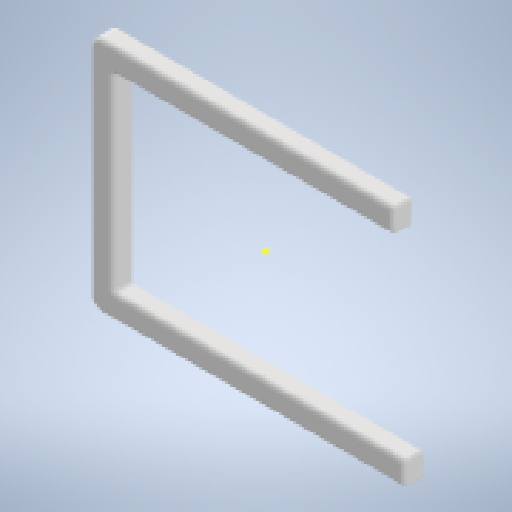
# Autodesk Inventor part: Top_Left
Saved by Autodesk Inventor 2023 (Build 270158000, 158)
## iProperties
Created: 2022-11-13
Part Number: Top_Left
Material: Generic
Document SubType Name: Modeling
Designer: reide
Density: 1 g/cm^3
Appearance: Default
Author: reide
Autodesk Inventor part; units mm, degrees
ref_plane "YZ Plane" through (0, 0, 0) normal (1, 0, 0) x (0, 1, 0)
ref_plane "XZ Plane" through (0, 0, 0) normal (0, 1, 0) x (-1, 0, 0)
ref_plane "XY Plane" through (0, 0, 0) normal (0, 0, 1) x (1, 0, 0)
sketch "Sketch1" plane through (0, 0, 0) normal (0, 0, 1) x (1, 0, 0)
  line L0 (44.2692, 42.6) -> (44.2692, 40.35) projected
  arc A0 (44.2692, 40.35) -> (45.2692, 39.35) centre (45.2692, 40.35) ccw projected
  line L1 (45.2692, 39.35) -> (59.7692, 39.35) projected
  arc A1 (59.7692, 39.35) -> (60.7692, 40.35) centre (59.7692, 40.35) ccw projected
  line L2 (60.7692, 40.35) -> (60.7692, 48.35) projected
  arc A2 (60.7692, 48.35) -> (59.7692, 49.35) centre (59.7692, 48.35) ccw projected
  line L3 (59.7692, 49.35) -> (-60.5312, 49.35) projected
  arc A3 (-60.5312, 49.35) -> (-65.5312, 44.35) centre (-60.5312, 44.35) ccw projected
  line L4 (-65.5312, 44.35) -> (-65.5312, -44.35) projected
  arc A4 (-65.5312, -44.35) -> (-60.5312, -49.35) centre (-60.5312, -44.35) ccw projected
  line L5 (-60.5312, -49.35) -> (64.5312, -49.35) projected
  arc A5 (64.5312, -49.35) -> (65.5312, -48.35) centre (64.5312, -48.35) ccw projected
  line L6 (65.5312, -48.35) -> (65.5312, -40.35) projected
  arc A6 (65.5312, -40.35) -> (64.5312, -39.35) centre (64.5312, -40.35) ccw projected
  line L7 (64.5312, -39.35) -> (49.5062, -39.35) projected
  line L8 (49.5062, -39.35) -> (49.5062, -41.65) projected
  arc A7 (48.5062, -42.65) -> (49.5062, -41.65) centre (48.5062, -41.65) ccw projected
  line L9 (48.5062, -42.65) -> (29.9062, -42.65) projected
  arc A8 (28.9062, -41.65) -> (29.9062, -42.65) centre (29.9062, -41.65) ccw projected
  line L10 (28.9062, -41.65) -> (28.9062, -39.35) projected
  line L11 (28.9062, -39.35) -> (-18.4058, -39.35) projected
  line L12 (-18.4058, -39.35) -> (-18.4058, -41.65) projected
  arc A9 (-19.4058, -42.65) -> (-18.4058, -41.65) centre (-19.4058, -41.65) ccw projected
  line L13 (-19.4058, -42.65) -> (-38.0058, -42.65) projected
  arc A10 (-39.0058, -41.65) -> (-38.0058, -42.65) centre (-38.0058, -41.65) ccw projected
  line L14 (-39.0058, -41.65) -> (-39.0058, -39.35) projected
  line L15 (-39.0058, -39.35) -> (-54.5312, -39.35) projected
  arc A11 (-55.5312, -38.35) -> (-54.5312, -39.35) centre (-54.5312, -38.35) ccw projected
  line L16 (-55.5312, -38.35) -> (-55.5312, -17.1) projected
  arc A12 (-55.5312, -17.1) -> (-56.5312, -16.1) centre (-56.5312, -17.1) ccw projected
  line L17 (-56.5312, -16.1) -> (-58.7812, -16.1) projected
  arc A13 (-59.7812, -15.1) -> (-58.7812, -16.1) centre (-58.7812, -15.1) ccw projected
  line L18 (-59.7812, -15.1) -> (-59.7812, -4.1) projected
  arc A14 (-58.7812, -3.1) -> (-59.7812, -4.1) centre (-58.7812, -4.1) ccw projected
  line L19 (-58.7812, -3.1) -> (-56.5312, -3.1) projected
  arc A15 (-56.5312, -3.1) -> (-55.5312, -2.1) centre (-56.5312, -2.1) ccw projected
  line L20 (-55.5312, -2.1) -> (-55.5312, 2.225) projected
  line L21 (-55.5312, 2.225) -> (-57.8308, 2.225) projected
  arc A16 (-58.8308, 3.225) -> (-57.8308, 2.225) centre (-57.8308, 3.225) ccw projected
  line L22 (-58.8308, 3.225) -> (-58.8308, 21.825) projected
  arc A17 (-57.8308, 22.825) -> (-58.8308, 21.825) centre (-57.8308, 21.825) ccw projected
  line L23 (-57.8308, 22.825) -> (-55.5312, 22.825) projected
  line L24 (-55.5312, 22.825) -> (-55.5312, 38.35) projected
  arc A18 (-54.5312, 39.35) -> (-55.5312, 38.35) centre (-54.5312, 38.35) ccw projected
  line L25 (-54.5312, 39.35) -> (-39.0058, 39.35) projected
  line L26 (-39.0058, 39.35) -> (-39.0058, 41.65) projected
  arc A19 (-38.0058, 42.65) -> (-39.0058, 41.65) centre (-38.0058, 41.65) ccw projected
  line L27 (-38.0058, 42.65) -> (-19.4058, 42.65) projected
  arc A20 (-18.4058, 41.65) -> (-19.4058, 42.65) centre (-19.4058, 41.65) ccw projected
  line L28 (-18.4058, 41.65) -> (-18.4058, 39.35) projected
  line L29 (-18.4058, 39.35) -> (0.3317, 39.35) projected
  line L30 (0.3317, 39.35) -> (0.3317, 41.65) projected
  arc A21 (1.3317, 42.65) -> (0.3317, 41.65) centre (1.3317, 41.65) ccw projected
  line L31 (1.3317, 42.65) -> (19.9317, 42.65) projected
  arc A22 (20.9317, 41.65) -> (19.9317, 42.65) centre (19.9317, 41.65) ccw projected
  line L32 (20.9317, 41.65) -> (20.9317, 39.35) projected
  line L33 (20.9317, 39.35) -> (25.2692, 39.35) projected
  arc A23 (25.2692, 39.35) -> (26.2692, 40.35) centre (25.2692, 40.35) ccw projected
  line L34 (26.2692, 40.35) -> (26.2692, 42.35) projected
  arc A24 (25.2692, 41.35) -> (26.2692, 42.35) centre (25.2692, 42.35) ccw projected
  line L35 (25.2692, 41.35) -> (21.9317, 41.35) projected
  arc A25 (20.9317, 42.35) -> (21.9317, 41.35) centre (21.9317, 42.35) ccw projected
  line L36 (20.9317, 44.2959) -> (20.9317, 42.35) projected
  ellipse E0 centre (21.9317, 44.2959) end of major axis (21.9317, 43.2418) minor radius 1 (21.9317, 45.35) -> (20.9317, 44.2959) ccw projected
  line L37 (21.9317, 45.35) -> (34.9317, 45.35) projected
  ellipse E1 centre (34.9317, 44.2959) end of major axis (34.9317, 43.2418) minor radius 1 (35.9207, 44.452) -> (34.9317, 45.35) ccw projected
  arc A26 (34.9317, 43.6) -> (35.9207, 44.452) centre (34.9317, 44.6) ccw projected
  line L38 (34.9317, 43.6) -> (43.2692, 43.6) projected
  arc A27 (44.2692, 42.6) -> (43.2692, 43.6) centre (43.2692, 42.6) ccw projected
  arc A28 (-39.0058, -42.35) -> (-40.0058, -41.35) centre (-40.0058, -42.35) ccw projected
  line L39 (-39.0058, -44.2959) -> (-39.0058, -42.35) projected
  ellipse E2 centre (-40.0058, -44.2959) end of major axis (-40.0058, -43.2418) minor radius 1 (-40.0058, -45.35) -> (-39.0058, -44.2959) ccw projected
  line L40 (-40.0058, -45.35) -> (-53.0057, -45.35) projected
  ellipse E3 centre (-53.0057, -44.2959) end of major axis (-53.0057, -43.2418) minor radius 1 (-54.0057, -44.2959) -> (-53.0057, -45.35) ccw projected
  line L41 (-54.0057, -42.35) -> (-54.0057, -44.2959) projected
  arc A29 (-53.0057, -41.35) -> (-54.0057, -42.35) centre (-53.0057, -42.35) ccw projected
  line L42 (-53.0057, -41.35) -> (-40.0058, -41.35) projected
  circle A30 centre (55.7692, 44.35) radius 2.125 projected
  circle A31 centre (-60.5312, 44.35) radius 2.125 projected
  circle A32 centre (-60.5312, -44.35) radius 2.125 projected
  circle A33 centre (60.5312, -44.35) radius 2.125 projected
  line L43 (-40.0058, 41.35) -> (-53.0058, 41.35) projected
  arc A34 (-54.0058, 42.35) -> (-53.0058, 41.35) centre (-53.0058, 42.35) ccw projected
  line L44 (-54.0058, 44.2959) -> (-54.0058, 42.35) projected
  ellipse E4 centre (-53.0058, 44.2959) end of major axis (-53.0058, 43.2418) minor radius 1 (-53.0058, 45.35) -> (-54.0058, 44.2959) ccw projected
  line L45 (-53.0058, 45.35) -> (-40.0058, 45.35) projected
  ellipse E5 centre (-40.0058, 44.2959) end of major axis (-40.0058, 43.2418) minor radius 1 (-39.0058, 44.2959) -> (-40.0058, 45.35) ccw projected
  line L46 (-39.0058, 42.35) -> (-39.0058, 44.2959) projected
  arc A35 (-40.0058, 41.35) -> (-39.0058, 42.35) centre (-40.0058, 42.35) ccw projected
  arc A36 (28.9062, -42.35) -> (27.9062, -41.35) centre (27.9062, -42.35) ccw projected
  line L47 (28.9062, -44.2959) -> (28.9062, -42.35) projected
  ellipse E6 centre (27.9062, -44.2959) end of major axis (27.9062, -43.2418) minor radius 1 (27.9063, -45.35) -> (28.9062, -44.2959) ccw projected
  line L48 (27.9063, -45.35) -> (14.9063, -45.35) projected
  ellipse E7 centre (14.9063, -44.2959) end of major axis (14.9063, -43.2418) minor radius 1 (13.9063, -44.2959) -> (14.9063, -45.35) ccw projected
  line L49 (13.9063, -42.35) -> (13.9063, -44.2959) projected
  arc A37 (14.9063, -41.35) -> (13.9063, -42.35) centre (14.9063, -42.35) ccw projected
  line L50 (14.9063, -41.35) -> (27.9062, -41.35) projected
  line L51 (-39.0058, 39.35) -> (45.2692, 39.35)
  line L52 (-55.5312, 22.825) -> (-55.5312, -17.1)
  line L53 (-39.0058, -39.35) -> (49.5062, -39.35)
  point P0 (0, 0)
  point P1 (-55.5312, 2.225)
  constraints: 6 end point, 2 perpendicular, 1 horizontal, 8 other
extrude "Extrusion1" add sketch "Sketch1" along normal blind 7.5 contours A27 L38 A26 E1 L37 E0 L36 A25 L35 A24 L34 A23 L33 L32 A22 L31 A21 L30 L29 L28 A20 L27 A19 L26 L25 A18 L24 L23 A17 L22 A16 L21 L20 A15 L19 A14 L18 A13 L17 A12 L16 A11 L15 L14 A10 L13 A9 L12 L11 L10 A8 L9 A7 L8 L7 A6 L6 A5 L5 A4 L4 A3 L3 A2 L2 A1 L1 A0 L0 | L0 A0 L51 A23 L34 A24 L35 A25 L36 E0 L37 E1 A26 L38 A27 | L51 L30 A21 L31 A22 L32 | L51 L26 A19 L27 A20 L28 | L52 L21 A16 L22 A17 L23 | L52 A12 L17 A13 L18 A14 L19 A15 | L8 A7 L9 A8 L10 L53 | L53 L12 A9 L13 A10 L14 | L39 E2 L40 E3 L41 A29 L42 A28 | A30 | A31 | A32 | A33 | L43 A34 L44 E4 L45 E5 L46 A35 | L47 E6 L48 E7 L49 A37 L50 A36
fillet "Fillet1" radius 2 30 edges at (65.2384, -49.0571, 7.5) (65.5312, -44.35, 7.5) (65.2384, -39.6429, 7.5) (-46.7685, -39.35, 7.5) (-28.7058, -39.35, 7.5) (5.2502, -39.35, 7.5) (39.2062, -39.35, 7.5) (57.0187, -39.35, 7.5) (-55.2384, -39.0571, 7.5) (-55.5312, 30.5875, 7.5) (-55.5312, 12.525, 7.5) (-55.5312, 0.0625, 7.5) (-55.5312, -9.6, 7.5) (-55.5312, -27.725, 7.5) (-55.2384, 39.0571, 7.5) (52.5192, 39.35, 7.5) (35.2692, 39.35, 7.5) (23.1005, 39.35, 7.5) (10.6317, 39.35, 7.5) (-9.037, 39.35, 7.5) (-28.7058, 39.35, 7.5) (-46.7685, 39.35, 7.5) (60.4764, 39.6429, 7.5) (60.7692, 44.35, 7.5) (60.4764, 49.0571, 7.5) (-0.381, 49.35, 7.5) (-64.0668, 47.8855, 7.5) (-65.5312, 0, 7.5) (-64.0668, -47.8855, 7.5) (2, -49.35, 7.5)
sketch "Sketch3" plane through (65.5312, -48.35, 0) normal (1, 0, 0) x (0, 0, -1)
  line L0 (0, -1) -> (-5.5, -1) projected
  line L1 (0, 9) -> (-5.5, 9) projected
  line L2 (0, 9) -> (0, 7)
  line L3 (0, 7) -> (-3, 7)
  line L4 (-3, 7) -> (-3, 1.7)
  line L5 (0, 7) -> (0, 2.7)
  line L6 (0, 2.7) -> (-3, 1.7)
  line L7 (0, 48.35) -> (-9, 48.35)
  line L8 (0, 97.7) -> (-5.5, 97.7)
  line L9 (0, 87.7) -> (-5.5, 87.7)
  line L10 (0, 87.7) -> (0, 89.7)
  line L11 (0, 89.7) -> (-3, 89.7)
  line L12 (-3, 89.7) -> (-3, 95)
  line L13 (0, 89.7) -> (0, 94)
  line L14 (0, 90.575) -> (0, 94.825)
  line L15 (0, 94) -> (-3, 95)
  point P0 (0, 6.125)
  point P1 (0, 1.875)
  dimension "d5" = 2
  dimension "d6" = 3
  dimension "d7" = 5.3
  dimension "d8" = 4.3
  constraints: 28 end point, 10 symmetric about line, 2 vertical, 1 horizontal, 1 perpendicular, 1 point on line
  measures "d5" distance of L1.start L2.end
  measures "d6" distance of L2.end L3.end
  measures "d7" distance of L3.end L4.end
  measures "d8" distance of L2.end L5.end
extrude "Extrusion3" cut sketch "Sketch3" against normal up to surface (131.0625 mm away)
sketch "Sketch4" plane through (0, 0, 0) normal (0, 0, -1) x (-1, 0, 0)
  point P0 (0, 0)
sketch "Sketch5" plane through (0, 0, 0) normal (0, 0, -1) x (-1, 0, 0)
  line L0 (54.0057, -42.35) -> (54.0057, -44.2959) projected
  line L1 (39.0058, -44.2959) -> (39.0058, -42.35) projected
  line L2 (-28.9062, -44.2959) -> (-28.9062, -42.35) projected
  line L3 (-13.9063, -42.35) -> (-13.9063, -44.2959) projected
  line L4 (-44.2692, 42.6) -> (-44.2692, 40.35) projected
  arc A0 (-45.2692, 39.35) -> (-44.2692, 40.35) centre (-45.2692, 40.35) ccw projected
  line L5 (-45.2692, 39.35) -> (-59.7692, 39.35) projected
  arc A1 (-60.7692, 40.35) -> (-59.7692, 39.35) centre (-59.7692, 40.35) ccw projected
  line L6 (-60.7692, 40.35) -> (-60.7692, 48.35) projected
  arc A2 (-59.7692, 49.35) -> (-60.7692, 48.35) centre (-59.7692, 48.35) ccw projected
  line L7 (-59.7692, 49.35) -> (60.5312, 49.35) projected
  arc A3 (65.5312, 44.35) -> (60.5312, 49.35) centre (60.5312, 44.35) ccw projected
  line L8 (65.5312, 44.35) -> (65.5312, -44.35) projected
  arc A4 (60.5312, -49.35) -> (65.5312, -44.35) centre (60.5312, -44.35) ccw projected
  line L9 (60.5312, -49.35) -> (-64.5312, -49.35) projected
  arc A5 (-65.5312, -48.35) -> (-64.5312, -49.35) centre (-64.5312, -48.35) ccw projected
  line L10 (-65.5312, -48.35) -> (-65.5312, -40.35) projected
  arc A6 (-64.5312, -39.35) -> (-65.5312, -40.35) centre (-64.5312, -40.35) ccw projected
  line L11 (-64.5312, -39.35) -> (-49.5062, -39.35) projected
  line L12 (-49.5062, -39.35) -> (-49.5062, -41.65) projected
  arc A7 (-49.5062, -41.65) -> (-48.5062, -42.65) centre (-48.5062, -41.65) ccw projected
  line L13 (-48.5062, -42.65) -> (-29.9062, -42.65) projected
  arc A8 (-29.9062, -42.65) -> (-28.9062, -41.65) centre (-29.9062, -41.65) ccw projected
  line L14 (-28.9062, -41.65) -> (-28.9062, -39.35) projected
  line L15 (-28.9062, -39.35) -> (18.4058, -39.35) projected
  line L16 (18.4058, -39.35) -> (18.4058, -41.65) projected
  arc A9 (18.4058, -41.65) -> (19.4058, -42.65) centre (19.4058, -41.65) ccw projected
  line L17 (19.4058, -42.65) -> (38.0058, -42.65) projected
  arc A10 (38.0058, -42.65) -> (39.0058, -41.65) centre (38.0058, -41.65) ccw projected
  line L18 (39.0058, -41.65) -> (39.0058, -39.35) projected
  line L19 (39.0058, -39.35) -> (54.5312, -39.35) projected
  arc A11 (54.5312, -39.35) -> (55.5312, -38.35) centre (54.5312, -38.35) ccw projected
  line L20 (55.5312, -38.35) -> (55.5312, -17.1) projected
  arc A12 (56.5312, -16.1) -> (55.5312, -17.1) centre (56.5312, -17.1) ccw projected
  line L21 (56.5312, -16.1) -> (58.7812, -16.1) projected
  arc A13 (58.7812, -16.1) -> (59.7812, -15.1) centre (58.7812, -15.1) ccw projected
  line L22 (59.7812, -15.1) -> (59.7812, -4.1) projected
  arc A14 (59.7812, -4.1) -> (58.7812, -3.1) centre (58.7812, -4.1) ccw projected
  line L23 (58.7812, -3.1) -> (56.5312, -3.1) projected
  arc A15 (55.5312, -2.1) -> (56.5312, -3.1) centre (56.5312, -2.1) ccw projected
  line L24 (55.5312, -2.1) -> (55.5312, 2.225) projected
  line L25 (55.5312, 2.225) -> (57.8308, 2.225) projected
  arc A16 (57.8308, 2.225) -> (58.8308, 3.225) centre (57.8308, 3.225) ccw projected
  line L26 (58.8308, 3.225) -> (58.8308, 21.825) projected
  arc A17 (58.8308, 21.825) -> (57.8308, 22.825) centre (57.8308, 21.825) ccw projected
  line L27 (57.8308, 22.825) -> (55.5312, 22.825) projected
  line L28 (55.5312, 22.825) -> (55.5312, 38.35) projected
  arc A18 (55.5312, 38.35) -> (54.5312, 39.35) centre (54.5312, 38.35) ccw projected
  line L29 (54.5312, 39.35) -> (39.0058, 39.35) projected
  line L30 (39.0058, 39.35) -> (39.0058, 41.65) projected
  arc A19 (39.0058, 41.65) -> (38.0058, 42.65) centre (38.0058, 41.65) ccw projected
  line L31 (38.0058, 42.65) -> (19.4058, 42.65) projected
  arc A20 (19.4058, 42.65) -> (18.4058, 41.65) centre (19.4058, 41.65) ccw projected
  line L32 (18.4058, 41.65) -> (18.4058, 39.35) projected
  line L33 (18.4058, 39.35) -> (-0.3317, 39.35) projected
  line L34 (-0.3317, 39.35) -> (-0.3317, 41.65) projected
  arc A21 (-0.3317, 41.65) -> (-1.3317, 42.65) centre (-1.3317, 41.65) ccw projected
  line L35 (-1.3317, 42.65) -> (-19.9317, 42.65) projected
  arc A22 (-19.9317, 42.65) -> (-20.9317, 41.65) centre (-19.9317, 41.65) ccw projected
  line L36 (-20.9317, 41.65) -> (-20.9317, 39.35) projected
  line L37 (-20.9317, 39.35) -> (-25.2692, 39.35) projected
  arc A23 (-26.2692, 40.35) -> (-25.2692, 39.35) centre (-25.2692, 40.35) ccw projected
  line L38 (-26.2692, 40.35) -> (-26.2692, 42.35) projected
  arc A24 (-26.2692, 42.35) -> (-25.2692, 41.35) centre (-25.2692, 42.35) ccw projected
  line L39 (-25.2692, 41.35) -> (-21.9317, 41.35) projected
  arc A25 (-21.9317, 41.35) -> (-20.9317, 42.35) centre (-21.9317, 42.35) ccw projected
  line L40 (-20.9317, 44.2959) -> (-20.9317, 42.35) projected
  ellipse E0 centre (-21.9317, 44.2959) end of major axis (-21.9317, 43.2418) minor radius 1 (-20.9317, 44.2959) -> (-21.9317, 45.35) ccw projected
  line L41 (-21.9317, 45.35) -> (-34.9317, 45.35) projected
  ellipse E1 centre (-34.9317, 44.2959) end of major axis (-34.9317, 43.2418) minor radius 1 (-34.9317, 45.35) -> (-35.9207, 44.452) ccw projected
  arc A26 (-35.9207, 44.452) -> (-34.9317, 43.6) centre (-34.9317, 44.6) ccw projected
  line L42 (-34.9317, 43.6) -> (-43.2692, 43.6) projected
  arc A27 (-43.2692, 43.6) -> (-44.2692, 42.6) centre (-43.2692, 42.6) ccw projected
  arc A28 (40.0058, -41.35) -> (39.0058, -42.35) centre (40.0058, -42.35) ccw projected
  line L43 (39.0058, -44.2959) -> (39.0058, -42.35) projected
  ellipse E2 centre (40.0058, -44.2959) end of major axis (40.0058, -43.2418) minor radius 1 (39.0058, -44.2959) -> (40.0058, -45.35) ccw projected
  line L44 (40.0058, -45.35) -> (53.0057, -45.35) projected
  ellipse E3 centre (53.0057, -44.2959) end of major axis (53.0057, -43.2418) minor radius 1 (53.0057, -45.35) -> (54.0057, -44.2959) ccw projected
  line L45 (54.0057, -42.35) -> (54.0057, -44.2959) projected
  arc A29 (54.0057, -42.35) -> (53.0057, -41.35) centre (53.0057, -42.35) ccw projected
  line L46 (53.0057, -41.35) -> (40.0058, -41.35) projected
  circle A30 centre (-55.7692, 44.35) radius 2.125 projected
  circle A31 centre (60.5312, 44.35) radius 2.125 projected
  circle A32 centre (60.5312, -44.35) radius 2.125 projected
  circle A33 centre (-60.5312, -44.35) radius 2.125 projected
  line L47 (40.0058, 41.35) -> (53.0058, 41.35) projected
  arc A34 (53.0058, 41.35) -> (54.0058, 42.35) centre (53.0058, 42.35) ccw projected
  line L48 (54.0058, 44.2959) -> (54.0058, 42.35) projected
  ellipse E4 centre (53.0058, 44.2959) end of major axis (53.0058, 43.2418) minor radius 1 (54.0058, 44.2959) -> (53.0058, 45.35) ccw projected
  line L49 (53.0058, 45.35) -> (40.0058, 45.35) projected
  ellipse E5 centre (40.0058, 44.2959) end of major axis (40.0058, 43.2418) minor radius 1 (40.0058, 45.35) -> (39.0058, 44.2959) ccw projected
  line L50 (39.0058, 42.35) -> (39.0058, 44.2959) projected
  arc A35 (39.0058, 42.35) -> (40.0058, 41.35) centre (40.0058, 42.35) ccw projected
  arc A36 (-27.9062, -41.35) -> (-28.9062, -42.35) centre (-27.9062, -42.35) ccw projected
  line L51 (-28.9062, -44.2959) -> (-28.9062, -42.35) projected
  ellipse E6 centre (-27.9062, -44.2959) end of major axis (-27.9062, -43.2418) minor radius 1 (-28.9062, -44.2959) -> (-27.9063, -45.35) ccw projected
  line L52 (-27.9063, -45.35) -> (-14.9063, -45.35) projected
  ellipse E7 centre (-14.9063, -44.2959) end of major axis (-14.9063, -43.2418) minor radius 1 (-14.9063, -45.35) -> (-13.9063, -44.2959) ccw projected
  line L53 (-13.9063, -42.35) -> (-13.9063, -44.2959) projected
  arc A37 (-13.9063, -42.35) -> (-14.9063, -41.35) centre (-14.9063, -42.35) ccw projected
  line L54 (-14.9063, -41.35) -> (-27.9062, -41.35) projected
  arc A38 (64.9708, -46.65) -> (65.5312, -44.35) centre (60.5312, -44.35) ccw projected
  line L55 (65.5312, -41.35) -> (65.5312, -44.35) projected
  line L56 (-65.5312, -41.35) -> (65.5312, -41.35) projected
  line L57 (-65.5312, -46.65) -> (-65.5312, -41.35) projected
  line L58 (-65.5312, -46.65) -> (64.9708, -46.65) projected
  line L59 (54.5312, -41.35) -> (-63.5312, -41.35) projected
  line L60 (54.0058, -46.65) -> (39.0058, -46.65)
  line L61 (39.0058, -46.65) -> (39.0058, -41.35)
  line L62 (39.0058, -41.35) -> (54.0058, -41.35)
  line L63 (54.0058, -41.35) -> (54.0058, -46.65)
  line L64 (39.0058, -46.65) -> (23.0058, -46.65)
  line L65 (23.0058, -46.65) -> (23.0058, -41.35)
  line L66 (23.0058, -41.35) -> (39.0058, -41.35)
  line L67 (39.0058, -41.35) -> (39.0058, -46.65)
  line L68 (-13.9063, -41.35) -> (-28.9062, -41.35)
  line L69 (-28.9062, -41.35) -> (-28.9063, -46.65)
  line L70 (-28.9063, -46.65) -> (-13.9063, -46.65)
  line L71 (-13.9063, -46.65) -> (-13.9063, -41.35)
  line L72 (-28.9062, -41.35) -> (-44.9063, -41.35)
  line L73 (-44.9063, -41.35) -> (-44.9063, -46.65)
  line L74 (-44.9063, -46.65) -> (-28.9063, -46.65)
  line L75 (-28.9063, -46.65) -> (-28.9062, -41.35)
  line L76 (-60.7692, 46.65) -> (64.9708, 46.65) projected
  line L77 (65.5312, 41.35) -> (-60.7692, 41.35) projected
  line L78 (-60.7692, 41.35) -> (65.5312, 41.35) projected
  line L79 (54.0058, 41.35) -> (39.0058, 41.35)
  line L80 (39.0058, 41.35) -> (39.0058, 46.65)
  line L81 (39.0058, 46.65) -> (54.0058, 46.65)
  line L82 (54.0058, 46.65) -> (54.0058, 41.35)
  line L83 (39.0058, 46.65) -> (23.0058, 46.65)
  line L84 (23.0058, 46.65) -> (23.0058, 41.35)
  line L85 (23.0058, 41.35) -> (39.0058, 41.35)
  line L86 (39.0058, 41.35) -> (39.0058, 46.65)
  line L87 (-20.9317, 41.35) -> (-35.9317, 41.35)
  line L88 (-35.9317, 41.35) -> (-35.9317, 46.65)
  line L89 (-35.9317, 46.65) -> (-20.9317, 46.65)
  line L90 (-20.9317, 46.65) -> (-20.9317, 41.35)
  line L91 (-35.9317, 41.35) -> (-51.9317, 41.35)
  line L92 (-51.9317, 41.35) -> (-51.9317, 46.65)
  line L93 (-51.9317, 46.65) -> (-35.9317, 46.65)
  line L94 (-35.9317, 46.65) -> (-35.9317, 41.35)
  point P0 (0, 0)
  point P1 (23.0058, 46.65)
  point P2 (-20.9317, 46.65)
  point P3 (54.0058, 46.65)
  point P4 (-65.5312, -46.65)
  point P5 (-13.9063, -46.65)
  point P6 (23.0058, -46.65)
  point P7 (64.9708, -46.65)
  dimension "d11" = 16
  dimension "d12" = 15
  dimension "d13" = 16
  dimension "d14" = 15
  dimension "d15" = 16
  constraints: 64 end point, 16 parallel, 15 point on line, 8 horizontal, 8 perpendicular, 8 other
  measures "d11" distance between parallel lines of L65 L67
  measures "d12" distance between parallel lines of L75 L71
  measures "d13" distance between parallel lines of L73 L69
  measures "d14" distance between parallel lines of L88 L90
  measures "d15" distance between parallel lines of L92 L94
extrude "Extrusion4" add sketch "Sketch5" against normal up to surface (3 mm away) contours L63 L56 L8 A4 L58 L0 | L58 L71 L3 L56 L16 A9 L17 L65 | L65 L17 A9 L16 L56 | L77 L82 L48 L76 A3 L8 | L58 L10 L56 L12 A7 L13 L73 | L13 A7 L12 L56 L73 | L84 L31 A20 L32 L77 L34 A21 L35 A22 L90 L40 L76 | L77 L32 A20 L31 L84 | L76 L92 L77 L6 | L77 L36 A22 L35 A21 L34 | A30 | A31 | A32 | A33
sketch "Sketch6" plane through (0, 0, 0) normal (0, 0, -1) x (-1, 0, 0)
  line L0 (-65.5312, -48.35) -> (-65.5312, -40.35) projected
  arc A0 (-65.5312, -48.35) -> (-64.5312, -49.35) centre (-64.5312, -48.35) ccw projected
  line L1 (60.5312, -49.35) -> (-64.5312, -49.35) projected
  arc A1 (60.5312, -49.35) -> (65.5312, -44.35) centre (60.5312, -44.35) ccw projected
  arc A2 (65.5312, 44.35) -> (60.5312, 49.35) centre (60.5312, 44.35) ccw projected
  line L2 (-59.7692, 49.35) -> (60.5312, 49.35) projected
  arc A3 (-59.7692, 49.35) -> (-60.7692, 48.35) centre (-59.7692, 48.35) ccw projected
  line L3 (-60.7692, 40.35) -> (-60.7692, 48.35) projected
  arc A4 (-60.7692, 40.35) -> (-59.7692, 39.35) centre (-59.7692, 40.35) ccw projected
  line L4 (54.5312, 39.35) -> (-59.7692, 39.35) projected
  arc A5 (55.5312, 38.35) -> (54.5312, 39.35) centre (54.5312, 38.35) ccw projected
  line L5 (55.5312, -38.35) -> (55.5312, 38.35) projected
  arc A6 (54.5312, -39.35) -> (55.5312, -38.35) centre (54.5312, -38.35) ccw projected
  line L6 (-64.5312, -39.35) -> (54.5312, -39.35) projected
  arc A7 (-64.5312, -39.35) -> (-65.5312, -40.35) centre (-64.5312, -40.35) ccw projected
  line L7 (-44.9063, -45.65) -> (-44.9063, -41.35) projected
  line L8 (-44.9063, -41.35) -> (-13.9063, -41.35) projected
  line L9 (-13.9063, -41.35) -> (-13.9063, -45.65) projected
  line L10 (-13.9063, -45.65) -> (-44.9063, -45.65) projected
  line L11 (-20.9317, 41.35) -> (-51.9317, 41.35) projected
  line L12 (-51.9317, 41.35) -> (-51.9317, 45.65) projected
  line L13 (-51.9317, 45.65) -> (-20.9317, 45.65) projected
  line L14 (-20.9317, 45.65) -> (-20.9317, 41.35) projected
  line L15 (54.0058, -41.35) -> (54.0058, -45.65) projected
  line L16 (54.0058, -45.65) -> (23.0058, -45.65) projected
  line L17 (23.0058, -45.65) -> (23.0058, -41.35) projected
  line L18 (23.0058, -41.35) -> (54.0058, -41.35) projected
  line L19 (23.0058, 41.35) -> (23.0058, 45.65) projected
  line L20 (23.0058, 45.65) -> (54.0058, 45.65) projected
  line L21 (54.0058, 45.65) -> (54.0058, 41.35) projected
  line L22 (54.0058, 41.35) -> (23.0058, 41.35) projected
  line L23 (-44.2692, 42.6) -> (-44.2692, 40.35) projected
  arc A8 (-45.2692, 39.35) -> (-44.2692, 40.35) centre (-45.2692, 40.35) ccw projected
  line L24 (-45.2692, 39.35) -> (-59.7692, 39.35) projected
  arc A9 (-60.7692, 40.35) -> (-59.7692, 39.35) centre (-59.7692, 40.35) ccw projected
  line L25 (-60.7692, 40.35) -> (-60.7692, 48.35) projected
  arc A10 (-59.7692, 49.35) -> (-60.7692, 48.35) centre (-59.7692, 48.35) ccw projected
  line L26 (-59.7692, 49.35) -> (60.5312, 49.35) projected
  arc A11 (65.5312, 44.35) -> (60.5312, 49.35) centre (60.5312, 44.35) ccw projected
  line L27 (65.5312, 44.35) -> (65.5312, -44.35) projected
  arc A12 (60.5312, -49.35) -> (65.5312, -44.35) centre (60.5312, -44.35) ccw projected
  line L28 (60.5312, -49.35) -> (-64.5312, -49.35) projected
  arc A13 (-65.5312, -48.35) -> (-64.5312, -49.35) centre (-64.5312, -48.35) ccw projected
  line L29 (-65.5312, -48.35) -> (-65.5312, -40.35) projected
  arc A14 (-64.5312, -39.35) -> (-65.5312, -40.35) centre (-64.5312, -40.35) ccw projected
  line L30 (-64.5312, -39.35) -> (-49.5062, -39.35) projected
  line L31 (-49.5062, -39.35) -> (-49.5062, -41.65) projected
  arc A15 (-49.5062, -41.65) -> (-48.5062, -42.65) centre (-48.5062, -41.65) ccw projected
  line L32 (-48.5062, -42.65) -> (-29.9062, -42.65) projected
  arc A16 (-29.9062, -42.65) -> (-28.9062, -41.65) centre (-29.9062, -41.65) ccw projected
  line L33 (-28.9062, -41.65) -> (-28.9062, -39.35) projected
  line L34 (-28.9062, -39.35) -> (18.4058, -39.35) projected
  line L35 (18.4058, -39.35) -> (18.4058, -41.65) projected
  arc A17 (18.4058, -41.65) -> (19.4058, -42.65) centre (19.4058, -41.65) ccw projected
  line L36 (19.4058, -42.65) -> (38.0058, -42.65) projected
  arc A18 (38.0058, -42.65) -> (39.0058, -41.65) centre (38.0058, -41.65) ccw projected
  line L37 (39.0058, -41.65) -> (39.0058, -39.35) projected
  line L38 (39.0058, -39.35) -> (54.5312, -39.35) projected
  arc A19 (54.5312, -39.35) -> (55.5312, -38.35) centre (54.5312, -38.35) ccw projected
  line L39 (55.5312, -38.35) -> (55.5312, -17.1) projected
  arc A20 (56.5312, -16.1) -> (55.5312, -17.1) centre (56.5312, -17.1) ccw projected
  line L40 (56.5312, -16.1) -> (58.7812, -16.1) projected
  arc A21 (58.7812, -16.1) -> (59.7812, -15.1) centre (58.7812, -15.1) ccw projected
  line L41 (59.7812, -15.1) -> (59.7812, -4.1) projected
  arc A22 (59.7812, -4.1) -> (58.7812, -3.1) centre (58.7812, -4.1) ccw projected
  line L42 (58.7812, -3.1) -> (56.5312, -3.1) projected
  arc A23 (55.5312, -2.1) -> (56.5312, -3.1) centre (56.5312, -2.1) ccw projected
  line L43 (55.5312, -2.1) -> (55.5312, 2.225) projected
  line L44 (55.5312, 2.225) -> (57.8308, 2.225) projected
  arc A24 (57.8308, 2.225) -> (58.8308, 3.225) centre (57.8308, 3.225) ccw projected
  line L45 (58.8308, 3.225) -> (58.8308, 21.825) projected
  arc A25 (58.8308, 21.825) -> (57.8308, 22.825) centre (57.8308, 21.825) ccw projected
  line L46 (57.8308, 22.825) -> (55.5312, 22.825) projected
  line L47 (55.5312, 22.825) -> (55.5312, 38.35) projected
  arc A26 (55.5312, 38.35) -> (54.5312, 39.35) centre (54.5312, 38.35) ccw projected
  line L48 (54.5312, 39.35) -> (39.0058, 39.35) projected
  line L49 (39.0058, 39.35) -> (39.0058, 41.65) projected
  arc A27 (39.0058, 41.65) -> (38.0058, 42.65) centre (38.0058, 41.65) ccw projected
  line L50 (38.0058, 42.65) -> (19.4058, 42.65) projected
  arc A28 (19.4058, 42.65) -> (18.4058, 41.65) centre (19.4058, 41.65) ccw projected
  line L51 (18.4058, 41.65) -> (18.4058, 39.35) projected
  line L52 (18.4058, 39.35) -> (-0.3317, 39.35) projected
  line L53 (-0.3317, 39.35) -> (-0.3317, 41.65) projected
  arc A29 (-0.3317, 41.65) -> (-1.3317, 42.65) centre (-1.3317, 41.65) ccw projected
  line L54 (-1.3317, 42.65) -> (-19.9317, 42.65) projected
  arc A30 (-19.9317, 42.65) -> (-20.9317, 41.65) centre (-19.9317, 41.65) ccw projected
  line L55 (-20.9317, 41.65) -> (-20.9317, 39.35) projected
  line L56 (-20.9317, 39.35) -> (-25.2692, 39.35) projected
  arc A31 (-26.2692, 40.35) -> (-25.2692, 39.35) centre (-25.2692, 40.35) ccw projected
  line L57 (-26.2692, 40.35) -> (-26.2692, 42.35) projected
  arc A32 (-26.2692, 42.35) -> (-25.2692, 41.35) centre (-25.2692, 42.35) ccw projected
  line L58 (-25.2692, 41.35) -> (-21.9317, 41.35) projected
  arc A33 (-21.9317, 41.35) -> (-20.9317, 42.35) centre (-21.9317, 42.35) ccw projected
  line L59 (-20.9317, 44.2959) -> (-20.9317, 42.35) projected
  ellipse E0 centre (-21.9317, 44.2959) end of major axis (-21.9317, 43.2418) minor radius 1 (-20.9317, 44.2959) -> (-21.9317, 45.35) ccw projected
  line L60 (-21.9317, 45.35) -> (-34.9317, 45.35) projected
  ellipse E1 centre (-34.9317, 44.2959) end of major axis (-34.9317, 43.2418) minor radius 1 (-34.9317, 45.35) -> (-35.9207, 44.452) ccw projected
  arc A34 (-35.9207, 44.452) -> (-34.9317, 43.6) centre (-34.9317, 44.6) ccw projected
  line L61 (-34.9317, 43.6) -> (-43.2692, 43.6) projected
  arc A35 (-43.2692, 43.6) -> (-44.2692, 42.6) centre (-43.2692, 42.6) ccw projected
  arc A36 (40.0058, -41.35) -> (39.0058, -42.35) centre (40.0058, -42.35) ccw projected
  line L62 (39.0058, -44.2959) -> (39.0058, -42.35) projected
  ellipse E2 centre (40.0058, -44.2959) end of major axis (40.0058, -43.2418) minor radius 1 (39.0058, -44.2959) -> (40.0058, -45.35) ccw projected
  line L63 (40.0058, -45.35) -> (53.0057, -45.35) projected
  ellipse E3 centre (53.0057, -44.2959) end of major axis (53.0057, -43.2418) minor radius 1 (53.0057, -45.35) -> (54.0057, -44.2959) ccw projected
  line L64 (54.0057, -42.35) -> (54.0057, -44.2959) projected
  arc A37 (54.0057, -42.35) -> (53.0057, -41.35) centre (53.0057, -42.35) ccw projected
  line L65 (53.0057, -41.35) -> (40.0058, -41.35) projected
  circle A38 centre (-55.7692, 44.35) radius 2.125 projected
  circle A39 centre (60.5312, 44.35) radius 2.125 projected
  circle A40 centre (60.5312, -44.35) radius 2.125 projected
  circle A41 centre (-60.5312, -44.35) radius 2.125 projected
  line L66 (40.0058, 41.35) -> (53.0058, 41.35) projected
  arc A42 (53.0058, 41.35) -> (54.0058, 42.35) centre (53.0058, 42.35) ccw projected
  line L67 (54.0058, 44.2959) -> (54.0058, 42.35) projected
  ellipse E4 centre (53.0058, 44.2959) end of major axis (53.0058, 43.2418) minor radius 1 (54.0058, 44.2959) -> (53.0058, 45.35) ccw projected
  line L68 (53.0058, 45.35) -> (40.0058, 45.35) projected
  ellipse E5 centre (40.0058, 44.2959) end of major axis (40.0058, 43.2418) minor radius 1 (40.0058, 45.35) -> (39.0058, 44.2959) ccw projected
  line L69 (39.0058, 42.35) -> (39.0058, 44.2959) projected
  arc A43 (39.0058, 42.35) -> (40.0058, 41.35) centre (40.0058, 42.35) ccw projected
  arc A44 (-27.9062, -41.35) -> (-28.9062, -42.35) centre (-27.9062, -42.35) ccw projected
  line L70 (-28.9062, -44.2959) -> (-28.9062, -42.35) projected
  ellipse E6 centre (-27.9062, -44.2959) end of major axis (-27.9062, -43.2418) minor radius 1 (-28.9062, -44.2959) -> (-27.9063, -45.35) ccw projected
  line L71 (-27.9063, -45.35) -> (-14.9063, -45.35) projected
  ellipse E7 centre (-14.9063, -44.2959) end of major axis (-14.9063, -43.2418) minor radius 1 (-14.9063, -45.35) -> (-13.9063, -44.2959) ccw projected
  line L72 (-13.9063, -42.35) -> (-13.9063, -44.2959) projected
  arc A45 (-13.9063, -42.35) -> (-14.9063, -41.35) centre (-14.9063, -42.35) ccw projected
  line L73 (-14.9063, -41.35) -> (-27.9062, -41.35) projected
  line L74 (39.0058, 41.35) -> (23.0058, 41.35)
  line L75 (23.0058, 41.35) -> (23.0058, 45.65)
  line L76 (23.0058, 45.65) -> (39.0058, 45.65)
  line L77 (39.0058, 45.65) -> (39.0058, 41.35)
  line L78 (-51.9317, 41.35) -> (-35.9317, 41.35)
  line L79 (-35.9317, 41.35) -> (-35.9317, 45.65)
  line L80 (-35.9317, 45.65) -> (-51.9317, 45.65)
  line L81 (-51.9317, 45.65) -> (-51.9317, 41.35)
  line L82 (23.0058, -41.35) -> (54.0058, -41.35) projected
  line L83 (39.0058, -41.35) -> (23.0058, -41.35)
  line L84 (23.0058, -41.35) -> (23.0058, -45.65)
  line L85 (23.0058, -45.65) -> (39.0058, -45.65)
  line L86 (39.0058, -45.65) -> (39.0058, -41.35)
  line L87 (-28.9062, -41.35) -> (-44.9063, -41.35)
  line L88 (-44.9063, -41.35) -> (-44.9063, -45.65)
  line L89 (-44.9063, -45.65) -> (-28.9062, -45.65)
  line L90 (-28.9062, -45.65) -> (-28.9062, -41.35)
  line L91 (-20.9317, 41.35) -> (-20.9317, 46.65) projected
  line L92 (-51.9317, 46.65) -> (-20.9317, 46.65) projected
  line L93 (-51.9317, 46.65) -> (-51.9317, 41.35) projected
  line L94 (-51.9317, 41.35) -> (-20.9317, 41.35) projected
  line L95 (23.0058, 46.65) -> (23.0058, 41.35) projected
  line L96 (23.0058, 41.35) -> (54.0058, 41.35) projected
  line L97 (54.0058, 41.35) -> (54.0058, 46.65) projected
  line L98 (23.0058, 46.65) -> (54.0058, 46.65) projected
  line L99 (-44.9063, -41.35) -> (-44.9063, -46.65) projected
  line L100 (-44.9063, -46.65) -> (-13.9063, -46.65) projected
  line L101 (-13.9063, -46.65) -> (-13.9063, -41.35) projected
  line L102 (-44.9063, -41.35) -> (-13.9063, -41.35) projected
  line L103 (54.0058, -46.65) -> (54.0058, -41.35) projected
  line L104 (23.0058, -41.35) -> (54.0058, -41.35) projected
  line L105 (23.0058, -41.35) -> (23.0058, -46.65) projected
  line L106 (23.0058, -46.65) -> (54.0058, -46.65) projected
  line L107 (39.0058, -46.65) -> (23.0058, -46.65)
  line L108 (23.0058, -46.65) -> (23.0058, -41.35)
  line L109 (23.0058, -41.35) -> (39.0058, -41.35)
  line L110 (39.0058, -41.35) -> (39.0058, -46.65)
  line L111 (-28.9062, -46.65) -> (-44.9063, -46.65)
  line L112 (-44.9063, -46.65) -> (-44.9063, -41.35)
  line L113 (-44.9063, -41.35) -> (-28.9062, -41.35)
  line L114 (-28.9062, -41.35) -> (-28.9062, -46.65)
  line L115 (-35.9317, 41.35) -> (-51.9317, 41.35)
  line L116 (-51.9317, 41.35) -> (-51.9317, 46.65)
  line L117 (-51.9317, 46.65) -> (-35.9317, 46.65)
  line L118 (-35.9317, 46.65) -> (-35.9317, 41.35)
  line L119 (39.0058, 41.35) -> (23.0058, 41.35)
  line L120 (23.0058, 41.35) -> (23.0058, 46.65)
  line L121 (23.0058, 46.65) -> (39.0058, 46.65)
  line L122 (39.0058, 46.65) -> (39.0058, 41.35)
  line L123 (65.5312, 44.35) -> (65.5312, -44.35) projected
  point P0 (0, 0)
  point P1 (39.0058, 46.65)
  point P2 (-35.9317, 46.65)
  point P3 (-28.9062, -45.65)
  point P4 (-28.9062, -42.35)
  dimension "d18" = 16
  constraints: 64 end point, 16 parallel, 9 point on line, 8 horizontal, 8 perpendicular, 8 other
  measures "d18" distance between parallel lines of L12 L79
extrude "Extrusion5" cut sketch "Sketch6" against normal up to surface (3 mm away) contours L33 A16 L32 L7 L8 | L90 L70 L10 L7 L32 A16 | L37 A18 L36 L17 L18 | L10 L114 L100 L99 | L86 L62 L16 L17 L36 A18 | L16 L110 L106 L105 | L23 A35 L61 L79 L11 | L11 L12 L13 L79 L61 A35 L23 | L93 L92 L118 L13 | L22 L19 L50 A27 L49 | A27 L50 L19 L20 L77 L69 | L95 L98 L122 L20
sketch "Sketch7" plane through (0, 0, 0) normal (0, 0, -1) x (-1, 0, 0)
  circle A0 centre (60.5312, -44.35) radius 2.125 projected
  circle A1 centre (-60.5312, -44.35) radius 2.125 projected
  circle A2 centre (-55.7692, 44.35) radius 2.125 projected
  circle A3 centre (60.5312, 44.35) radius 2.125 projected
  point P0 (0, 0)
extrude "Extrusion6" cut sketch "Sketch7" against normal blind 1.8
body "Solid1"
